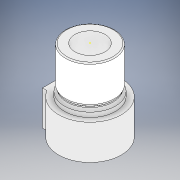
# Autodesk Inventor part: prednji deo
Saved by Autodesk Inventor 2019 (Build 230136000, 136)
## iProperties
Created: 2018-11-25
Part Number: prednji deo
Material: ABS Plastic
Document SubType Name: Modeling
Designer: aleks
Density: 1.06 g/cm^3
Appearance: Smooth - White
Author: aleks
Autodesk Inventor part; units mm, degrees
ref_plane "YZ Plane" through (0, 0, 0) normal (1, 0, 0) x (0, 1, 0)
ref_plane "XZ Plane" through (0, 0, 0) normal (0, 1, 0) x (-1, 0, 0)
ref_plane "XY Plane" through (0, 0, 0) normal (0, 0, 1) x (1, 0, 0)
sketch "Sketch1" plane through (0, 0, 0) normal (0, 1, 0) x (-1, 0, 0)
  arc A0 (11.5434, 7) -> (11.5434, -7) centre (0, 0) ccw
  line L0 (13.5, 0) -> (20.5, 0) construction
  line L1 (13.5, -7) -> (13.5, 7)
  line L2 (13.5, 7) -> (11.5434, 7)
  line L3 (13.5, -7) -> (11.5434, -7)
  dimension "d0" = 27
  dimension "d1" = 7
  dimension "d3" = 14
  constraints: 8 end point, 3 horizontal, 2 point on circle, 1 centre point, 1 coincident, 1 midpoint
  measures "d0" diameter of A0
  measures "d1" distance of L0.start L1.start
  measures "d3" distance of L1.start L1.end
extrude "Extrusion1" add sketch "Sketch1" along normal blind 15
sketch "Sketch2" plane through (0, 15, 0) normal (0, 1, 0) x (1, 0, 0)
  circle A0 centre (0, 0) radius 11
  dimension "d6" = 22
  constraints: 1 centre point, 1 coincident
  measures "d6" diameter of A0
extrude "Extrusion2" add sketch "Sketch2" along normal blind 2
sketch "Sketch3" plane through (0, 17, 0) normal (0, 1, 0) x (1, 0, 0)
  circle A0 centre (0, 0) radius 10
  dimension "d9" = 20
  constraints: 1 centre point, 1 coincident
  measures "d9" diameter of A0
extrude "Extrusion3" add sketch "Sketch3" along normal blind 2
sketch "Sketch4" plane through (0, 19, 0) normal (0, 1, 0) x (1, 0, 0)
  circle A0 centre (0, 0) radius 10.5
  dimension "d12" = 21
  constraints: 1 centre point, 1 coincident
  measures "d12" diameter of A0
extrude "Extrusion4" add sketch "Sketch4" along normal blind 16
fillet "Fillet1" radius 1 1 edges at (-10, 17, 0)
chamfer "Chamfer1" distance 0.5 angle 45 2 edges at (-10, 19, 0) (-10.5, 19, 0)
fillet "Fillet2" radius 0.5 1 edges at (-10.5, 35, 0)
thread "Thread1" size "M10x1" class "6g" standard "ISO Metric profile" full length
sketch "Sketch5" plane through (-13.5, 0, -7) normal (-1, 0, 0) x (0, 0, 1)
  point P0 (7, 0)
sketch "Sketch6" plane through (0, 0, 0) normal (0, -1, 0) x (1, 0, 0)
  circle A0 centre (0, 0) radius 7.5
  dimension "d22" = 15
  constraints: 1 centre point, 1 coincident
  measures "d22" diameter of A0
extrude "Extrusion5" cut sketch "Sketch6" against normal blind 25
sketch "Sketch7" plane through (-13.5, 0, -7) normal (-1, 0, 0) x (0, 0, 1)
  circle A0 centre (7, 7.5) radius 4.5
  point P0 (7, 0)
  dimension "d25" = 9
  constraints: 1 centre point
  measures "d25" diameter of A0
extrude "Extrusion6" cut sketch "Sketch7" against normal blind 18
thread "Thread2" size "M8x0.8" class "6H" standard "ISO Metric profile" full length
sketch "Sketch8" plane through (0, 35, 0) normal (0, 1, 0) x (1, 0, 0)
  circle A0 centre (0, 0) radius 6.5
  dimension "d30" = 13
  constraints: 1 centre point, 1 coincident
  measures "d30" diameter of A0
extrude "Extrusion7" cut sketch "Sketch8" against normal blind 18
sketch "Sketch9" plane through (0, 35, 0) normal (0, 1, 0) x (1, 0, 0)
  point P0 (0, 0)
body "Solid1"
